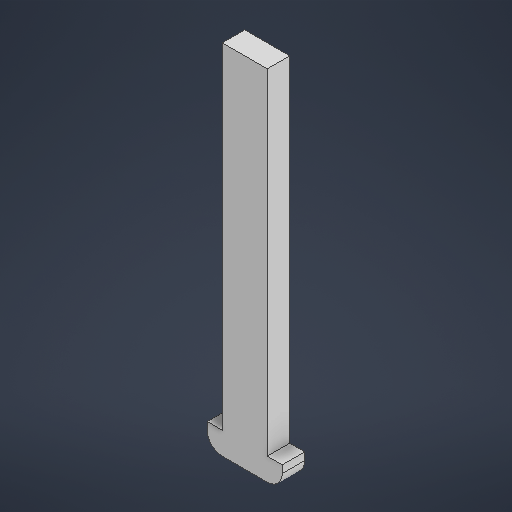
# Autodesk Inventor part: bolt
Saved by Autodesk Inventor 2025.3 (Build 293356030, 356C)
## iProperties
Created: 2025-10-01
Part Number: bolt
Material: 一般
Document SubType Name: Modeling
Designer: 陳泓任
Density: 1 g/cm^3
Appearance: 預設
Author: 陳泓任
Autodesk Inventor part; units mm, degrees
ref_plane "YZ Plane" through (0, 0, 0) normal (1, 0, 0) x (0, 1, 0)
ref_plane "XZ Plane" through (0, 0, 0) normal (0, 1, 0) x (-1, 0, 0)
ref_plane "XY Plane" through (0, 0, 0) normal (0, 0, 1) x (1, 0, 0)
sketch "草圖1" plane through (0, 0, 0) normal (0, 0, 1) x (1, 0, 0)
  line L0 (3, -20.85) -> (3, 23.85)
  line L1 (3, 23.85) -> (-3, 23.85)
  line L2 (-3, 23.85) -> (-3, -20.85)
  line L3 (-3, -23.85) -> (3, 23.85) construction
  line L4 (3, -23.85) -> (-3, 23.85) construction
  line L5 (5, -20.85) -> (5, -21.85)
  line L6 (3, -23.85) -> (-3, -23.85)
  line L7 (-5, -21.85) -> (-5, -20.85)
  line L8 (-5, -20.85) -> (-3, -20.85)
  line L9 (3, -20.85) -> (5, -20.85)
  line L10 (0, -16.0755) -> (0, 16.0755) construction
  arc A0 (-5, -21.85) -> (-3, -23.85) centre (-3, -21.85) ccw
  arc A1 (3, -23.85) -> (5, -21.85) centre (3, -21.85) ccw
  point P0 (0, 0)
  point P1 (5, -23.85)
  point P2 (-5, -23.85)
  dimension "d0" = 6
  dimension "d1" = 47.7
  dimension "d2" = 10
  dimension "d3" = 3
  dimension "d4" = 2
  constraints: 22 end point, 5 point on line, 4 parallel, 4 point on circle, 4 tangent, 3 horizontal, 3 midpoint, 2 centre point, 2 perpendicular, 1 collinear, 1 equal radius, 1 vertical, 2 other
  measures "d0" distance of L1.end L0.end
  measures "d1" distance of L4.start L0.end
  measures "d2" distance of point (5, -23.85) point (-5, -23.85)
  measures "d3" distance of L5.start point (5, -23.85)
  measures "d4" radius of A0
extrude "擠出1" add sketch "草圖1" along normal mid plane 3
